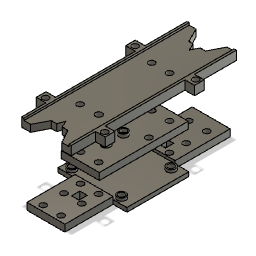
self balancing robot (Autodesk Fusion 360 design; units mm, degrees)
Autodesk Fusion 360 part; units mm, degrees
sketch "Sketch1" plane through (0, 0, 0) normal (0, 1, 0) x (1, 0, 0)
  circle A0 centre (-15, 25) radius 2.25
  circle A1 centre (-2, 25) radius 2.25
  circle A2 centre (-15, 40) radius 2.25
  circle A3 centre (-2, 40) radius 2.25
  line L0 (-11.7906, 20.4996) -> (-6.4075, 20.4996)
  line L1 (-6.4075, 20.4996) -> (-6.4075, 14.4996)
  line L2 (-6.4075, 14.4996) -> (-11.7906, 14.4996)
  line L3 (-11.7906, 14.4996) -> (-11.7906, 20.4996)
  circle A4 centre (-15, 12.9146) radius 2.25
  circle A5 centre (-2, 12.9014) radius 2.25
  circle A6 centre (7.0301, 5.1014) radius 2.25
  circle A7 centre (-28.9699, 5) radius 2.25
  circle A8 centre (-28.9697, -31) radius 2.25
  circle A9 centre (7.0301, -30.8986) radius 2.25
  circle A10 centre (-1.841, -50.8854) radius 2.25
  circle A11 centre (-14.841, -50.8854) radius 2.25
  line L4 (-10.4335, -49.7263) -> (-10.4335, -43.7263)
  circle A12 centre (-14.841, -38.8) radius 2.25
  circle A13 centre (-14.841, -65.8854) radius 2.25
  circle A14 centre (-1.841, -65.8854) radius 2.25
  circle A15 centre (-1.841, -38.6986) radius 2.25
  line L5 (-5.0503, -43.7263) -> (-5.0503, -49.7263)
  line L6 (-10.4335, -43.7263) -> (-5.0503, -43.7263)
  line L7 (-5.0503, -49.7263) -> (-10.4335, -49.7263)
  line L8 (-35, 50) -> (15, 50)
  line L9 (15, 50) -> (15, -70)
  line L10 (15, -70) -> (-35, -70)
  line L11 (-35, -70) -> (-35, 50)
  line L12 (5, 50) -> (5, 10)
  line L13 (5, 10) -> (15, 10)
  line L14 (-22.5777, 50) -> (-22.5777, 10)
  line L15 (-22.5777, 10) -> (-35, 10)
  line L16 (-22.5777, -70) -> (-22.5777, -35)
  line L17 (-22.5777, -35) -> (-35, -35)
  line L18 (5, -70) -> (5, -35)
  line L19 (5, -35) -> (15, -35)
  dimension "d1" = 4.5
  dimension "d2" = 4.5
  dimension "d3" = 4.5
  dimension "d4" = 4.5
  dimension "d5" = 15
  dimension "d6" = 13
  dimension "d7" = 13
  dimension "d9" = 6
  dimension "d10" = 4.5
  dimension "d11" = 4.5
  dimension "d15" = 4.5
  dimension "d16" = 4.5
  dimension "d17" = 4.5
  dimension "d18" = 4.5
  dimension "d19" = 36
  dimension "d20" = 36
  dimension "d21" = 36
  dimension "d22" = 36
  dimension "d23" = 4.5
  dimension "d24" = 4.5
  dimension "d25" = 4.5
  dimension "d26" = 4.5
  dimension "d27" = 15
  dimension "d28" = 13
  dimension "d29" = 13
  dimension "d30" = 6
  dimension "d31" = 4.5
  dimension "d32" = 4.5
  dimension "d33" = 7.8
  dimension "d34" = 7.8
  dimension "d35" = 13
  dimension "d36" = 13
  dimension "d37" = 12.0986
  dimension "d38" = 12.0854
  dimension "d39" = 7.9146
  dimension "d40" = 7.8
  dimension "d41" = 50
  dimension "d42" = 120
  dimension "d43" = 51.7146
  dimension "d44" = 51.6
  constraint horizontal L0
  constraint vertical L1
  constraint horizontal L2
  constraint vertical L3
  constraint horizontal L8
  constraint vertical L9
  constraint horizontal L10
  constraint vertical L11
  constraint coincident L8 L12.start
  constraint perpendicular L8 L12
  constraint coincident L9 L13.end
  constraint perpendicular L9 L13
  constraint coincident L8 L14.start
  constraint perpendicular L8 L14
  constraint coincident L11 L15.end
  constraint perpendicular L11 L15
  constraint coincident L10 L16.start
  constraint perpendicular L10 L16
  constraint coincident L11 L17.end
  constraint perpendicular L11 L17
  constraint perpendicular L13 L18
  constraint coincident L9 L19.end
  constraint perpendicular L9 L19
  measures "d1" diameter of A0
  measures "d2" diameter of A1
  measures "d3" diameter of A2
  measures "d4" diameter of A3
  measures "d5" distance of A0.centre A2.centre
  measures "d6" distance of A2.centre A3.centre
  measures "d7" distance of A0.centre A1.centre
  measures "d9" distance of L0.start L2.end
  measures "d10" diameter of A4
  measures "d11" diameter of A5
  measures "d15" diameter of A6
  measures "d16" diameter of A7
  measures "d17" diameter of A8
  measures "d18" diameter of A9
  measures "d19" horizontal distance of A6.centre A7.centre
  measures "d20" vertical distance of A7.centre A8.centre
  measures "d21" distance of A6.centre A9.centre
  measures "d22" distance of A8.centre A9.centre
  measures "d23" diameter of A10
  measures "d24" diameter of A11
  measures "d25" diameter of A14
  measures "d26" diameter of A13
  measures "d27" distance of A14.centre A10.centre
  measures "d28" distance of A14.centre A13.centre
  measures "d29" distance of A11.centre A10.centre
  measures "d30" distance of L5.end L5.start
  measures "d31" diameter of A15
  measures "d32" diameter of A12
  measures "d33" vertical distance of A5.centre A6.centre
  measures "d34" vertical distance of A9.centre A15.centre
  measures "d35" horizontal distance of A4.centre A5.centre
  measures "d36" horizontal distance of A15.centre A12.centre
  measures "d37" distance of A1.centre A5.centre
  measures "d38" distance of A12.centre A11.centre
  measures "d39" vertical distance of A4.centre A7.centre
  measures "d40" vertical distance of A8.centre A12.centre
  measures "d41" distance of L8.start L8.end
  measures "d42" distance of L8.start L10.end
  measures "d43" vertical distance of A4.centre A12.centre
  measures "d44" vertical distance of A5.centre A15.centre
extrude "Extrude1" add sketch "Sketch1" along normal blind 5 contours L8 L9 L10 L11 L12 L13 L14 L15 L16 L17 L18 L19 makes body 1
sketch "Sketch2" plane through (0, 5, 0) normal (0, 1, 0) x (-1, 0, 0)
  circle A0 centre (14.841, 65.8854) radius 2.25
  circle A1 centre (1.841, 38.6986) radius 2.25
  circle A2 centre (1.841, 65.8854) radius 2.25
  circle A3 centre (14.841, 38.8) radius 2.25
  line L0 (5.0503, 43.7263) -> (5.0503, 49.7263)
  line L1 (5.0503, 49.7263) -> (10.4335, 49.7263)
  line L2 (10.4335, 49.7263) -> (10.4335, 43.7263)
  line L3 (10.4335, 43.7263) -> (5.0503, 43.7263)
  circle A4 centre (-7.0301, -5.1014) radius 2.25
  circle A5 centre (28.9699, -5) radius 2.25
  circle A6 centre (28.9697, 31) radius 2.25
  circle A7 centre (-7.0301, 30.8986) radius 2.25
  circle A8 centre (1.841, 50.8854) radius 2.25
  circle A9 centre (14.841, 50.8854) radius 2.25
  circle A10 centre (2, -12.9014) radius 2.25
  circle A11 centre (15, -12.9146) radius 2.25
  circle A12 centre (2, -40) radius 2.25
  line L4 (6.4075, -14.4996) -> (11.7906, -14.4996)
  line L5 (11.7906, -14.4996) -> (11.7906, -20.4996)
  line L6 (11.7906, -20.4996) -> (6.4075, -20.4996)
  line L7 (6.4075, -20.4996) -> (6.4075, -14.4996)
  circle A13 centre (15, -40) radius 2.25
  circle A14 centre (2, -25) radius 2.25
  circle A15 centre (15, -25) radius 2.25
  line L8 (-5, 70) -> (-5, 35)
  line L9 (-5, 35) -> (-15, 35)
  line L10 (-15, 35) -> (-15, -10)
  line L11 (-15, -10) -> (-5, -10)
  line L12 (-5, -10) -> (-5, -50)
  line L13 (-5, -50) -> (22.5777, -50)
  line L14 (22.5777, -50) -> (22.5777, -10)
  line L15 (22.5777, -10) -> (35, -10)
  line L16 (35, -10) -> (35, 35)
  line L17 (35, 35) -> (22.5777, 35)
  line L18 (22.5777, 35) -> (22.5777, 70)
  line L19 (22.5777, 70) -> (-5, 70)
  line L20 (35, -10) -> (-15, -10)
  line L21 (-15, -10) -> (-15, 35)
  line L22 (-15, 35) -> (35, 35)
  line L23 (35, 35) -> (35, -10)
  circle A16 centre (28.9699, -5) radius 2.8072
  circle A17 centre (-7.0301, -5.1014) radius 3.2495
  circle A18 centre (-7.0301, 30.8986) radius 3.07
  circle A19 centre (28.9697, 31) radius 3.1528
  constraint horizontal L20
  constraint vertical L21
  constraint horizontal L22
  constraint vertical L23
  constraint coincident L9.end L10.start
  constraint coincident L15.end L16.start
  constraint concentric A5 A16
  constraint concentric A4 A17
  constraint concentric A7 A18
  constraint concentric A6 A19
extrude "Extrude2" cut sketch "Sketch2" against normal blind 2 contours L9 L10 L11 L15 L16 L17 L20 L21 L22 L23 bodies 1
sketch "Sketch3" plane through (0, 0, 0) normal (0, 0, 1) x (1, 0, 0)
sketch "Sketch4" plane through (0, 0, 0) normal (0, 1, 0) x (1, 0, 0)
  circle A0 centre (-15, 13) radius 2.25
  circle A1 centre (-2, 13) radius 2.25
  circle A2 centre (-14.819, -38.8151) radius 2.25
  circle A3 centre (-1.741, -38.7383) radius 2.25
  line L0 (-22.7552, 19.5423) -> (5, 19.5423)
  line L1 (5, 19.5423) -> (5, -45)
  line L2 (5, -45) -> (-22.7552, -45)
  line L3 (-22.7552, -45) -> (-22.7552, 19.5423)
  dimension "d49" = 4.5
  dimension "d50" = 4.5
  dimension "d51" = 4.5
  dimension "d52" = 4.5
  constraint horizontal L0
  constraint vertical L1
  constraint horizontal L2
  constraint vertical L3
  measures "d49" diameter of A0
  measures "d50" diameter of A1
  measures "d51" diameter of A2
  measures "d52" diameter of A3
extrude "Extrude3" add sketch "Sketch4" along normal blind 5 separate body makes body 2
move_body "Move1" bodies 2 to x (1, 0, 0) y (0, 1, 0) z (0, 0, 1) at (0, 20, 0)
sketch "Sketch5" plane through (0, 25, 0) normal (0, 1, 0) x (-1, 0, 0)
  circle A0 centre (14.819, 38.8151) radius 2.25
  circle A1 centre (1.741, 38.7383) radius 2.25
  circle A2 centre (2, -13) radius 2.25
  circle A3 centre (15, -13) radius 2.25
  line L0 (22.7552, 45) -> (-5, 45)
  line L1 (-5, 45) -> (-5, -19.5423)
  line L2 (-5, -19.5423) -> (22.7552, -19.5423)
  line L3 (22.7552, -19.5423) -> (22.7552, 45)
  circle A4 centre (10, 25) radius 2.25
  circle A5 centre (10, 12.5) radius 2.25
  circle A6 centre (10, 12.5) radius 3
  circle A7 centre (10, 25) radius 3
  circle A8 centre (-1, 5) radius 2.25
  dimension "d55" = 4.5
  dimension "d56" = 4.5
  dimension "d57" = 12.5
  dimension "d58" = 6
  dimension "d59" = 6
  dimension "d60" = 4.5
  constraint concentric A5 A6
  constraint concentric A4 A7
  measures "d55" diameter of A4
  measures "d56" diameter of A5
  measures "d57" distance of A4.centre A5.centre
  measures "d58" diameter of A6
  measures "d59" diameter of A7
  measures "d60" diameter of A8
extrude "Extrude4" add sketch "Sketch5" along normal blind 2.5 contours A6 | A7 bodies 2
extrude "Extrude5" cut sketch "Sketch5" against normal blind 5 contours A8 bodies 2
extrude "Extrude6" add sketch "Sketch5" against normal blind 5 contours A8 bodies 2
extrude "Extrude7" cut sketch "Sketch5" against normal blind 7 contours A8 bodies 2
sketch "Sketch6" plane through (0, 0, 0) normal (0, 1, 0) x (1, 0, 0)
  line L0 (-26.7355, 50.3207) -> (9.2645, 50.3207)
  line L1 (9.2645, 50.3207) -> (9.2645, -69.6793)
  line L2 (9.2645, -69.6793) -> (-26.7355, -69.6793)
  line L3 (-26.7355, -69.6793) -> (-26.7355, 50.3207)
  circle A0 centre (-14.9855, 13.0272) radius 2.25
  circle A1 centre (-2.0435, 13.0272) radius 2.25
  circle A2 centre (-15, -39) radius 2.25
  circle A3 centre (-1.6771, -38.6684) radius 2.4279
  line L4 (9.2645, 19.8475) -> (16.2645, 19.8475)
  line L5 (16.2645, 19.8475) -> (16.2645, 12.8475)
  line L6 (16.2645, 12.8475) -> (9.2645, 12.8475)
  line L7 (9.2645, 12.8475) -> (9.2645, 19.8475)
  line L8 (9.2645, -45.0475) -> (16.2645, -45.0475)
  line L9 (16.2645, -45.0475) -> (16.2645, -52.0475)
  line L10 (16.2645, -52.0475) -> (9.2645, -52.0475)
  line L11 (9.2645, -52.0475) -> (9.2645, -45.0475)
  line L12 (-26.7355, 19.8475) -> (-33.7355, 19.8475)
  line L13 (-33.7355, 19.8475) -> (-33.7355, 12.8475)
  line L14 (-33.7355, 12.8475) -> (-26.7355, 12.8475)
  line L15 (-26.7355, 12.8475) -> (-26.7355, 19.8475)
  line L16 (-26.7355, -45.0475) -> (-33.7355, -45.0475)
  line L17 (-33.7355, -45.0475) -> (-33.7355, -52.0475)
  line L18 (-33.7355, -52.0475) -> (-26.7355, -52.0475)
  line L19 (-26.7355, -52.0475) -> (-26.7355, -45.0475)
  circle A4 centre (-30, 16) radius 2.25
  circle A5 centre (13, 17) radius 2.25
  circle A6 centre (13, -49) radius 2.25
  circle A7 centre (-30, -49) radius 2.25
  line L20 (-20.1067, 50.3207) -> (-15, 40)
  line L21 (-15, 40) -> (-11.9429, 40)
  line L22 (-11.9429, 40) -> (-9.3767, 34.8138)
  line L23 (-9.3767, 34.8138) -> (-6.6947, 40)
  line L24 (-6.6947, 40) -> (-2.9044, 40)
  line L25 (-2.9044, 40) -> (2.4328, 50.3207)
  line L26 (-20.284, -69.6793) -> (-15.1632, -59.7773)
  line L27 (-15.1632, -59.7773) -> (-15.2822, -59.7773)
  line L28 (-9.3767, 34.8138) -> (-9.3767, -54.8804) construction
  line L29 (2.4328, 50.3207) -> (2.4328, -69.6793) construction
  line L30 (-2.9044, 40) -> (-2.9044, -60) construction
  line L31 (-15, 40) -> (-15.2227, -59.7773) construction
  line L32 (-15.2822, -59.7773) -> (-11.2248, -59.7773)
  line L33 (-11.2248, -59.7773) -> (-9.3767, -54.8804)
  line L34 (-9.3767, -54.8804) -> (-7.1721, -59.7773)
  line L35 (-7.1721, -59.7773) -> (-2.9044, -60)
  line L36 (-2.9044, -60) -> (2.4328, -69.6793)
  dimension "d69" = 36
  dimension "d70" = 120
  dimension "d71" = 4.5
  dimension "d72" = 4.5
  dimension "d73" = 4.5
  dimension "d74" = 7
  dimension "d75" = 7
  dimension "d76" = 7
  dimension "d77" = 7
  dimension "d78" = 7
  dimension "d79" = 7
  dimension "d80" = 7
  dimension "d81" = 7
  dimension "d82" = 4.5
  dimension "d83" = 4.5
  dimension "d84" = 4.5
  dimension "d85" = 4.5
  constraint horizontal L0
  constraint vertical L1
  constraint horizontal L2
  constraint vertical L3
  constraint horizontal L4
  constraint vertical L5
  constraint horizontal L6
  constraint vertical L7
  constraint coincident L1 L4.start
  constraint horizontal L8
  constraint vertical L9
  constraint horizontal L10
  constraint vertical L11
  constraint coincident L1 L8.start
  constraint horizontal L12
  constraint vertical L13
  constraint horizontal L14
  constraint vertical L15
  constraint coincident L3 L12.start
  constraint horizontal L16
  constraint vertical L17
  constraint horizontal L18
  constraint vertical L19
  constraint coincident L3 L16.start
  constraint coincident L0 L20.start
  constraint parallel L0 L21
  constraint parallel L20 L22
  constraint parallel L21 L24
  constraint coincident L0 L25.end
  constraint parallel L23 L25
  constraint coincident L2 L26.start
  constraint parallel L25 L26
  constraint parallel L2 L27
  constraint vertical L28
  constraint coincident L2 L29.end
  constraint perpendicular L2 L29
  constraint perpendicular L24 L30
  constraint midpoint L27 L31.end
  measures "d69" distance of L0.start L0.end
  measures "d70" distance of L0.start L2.end
  measures "d71" diameter of A0
  measures "d72" diameter of A1
  measures "d73" diameter of A2
  measures "d74" distance of L4.start L4.end
  measures "d75" distance of L4.start L6.end
  measures "d76" distance of L8.start L8.end
  measures "d77" distance of L8.start L10.end
  measures "d78" distance of L12.start L12.end
  measures "d79" distance of L12.start L14.end
  measures "d80" distance of L16.start L16.end
  measures "d81" distance of L16.start L18.end
  measures "d82" diameter of A4
  measures "d83" diameter of A5
  measures "d84" diameter of A6
  measures "d85" diameter of A7
extrude "Extrude8" add sketch "Sketch6" along normal blind 5 separate body contours L0 L1 L2 L3 L7 L11 L15 L19 L20 L21 L22 L23 L24 L25 L26 L32 L33 L34 L35 L36 | L3 L12 L13 L14 L15 | L3 L16 L17 L18 L19 | L1 L4 L5 L6 L7 | L1 L8 L9 L10 L11 makes body 3
sketch "Sketch7" plane through (0, 5, 0) normal (0, 1, 0) x (-1, 0, 0)
  circle A0 centre (30, 49) radius 2.25
  circle A1 centre (-13, -17) radius 2.25
  circle A2 centre (15, 39) radius 2.25
  circle A3 centre (-13, 49) radius 2.25
  circle A4 centre (1.6771, 38.6684) radius 2.4279
  circle A5 centre (30, -16) radius 2.25
  circle A6 centre (2.0435, -13.0272) radius 2.25
  circle A7 centre (14.9855, -13.0272) radius 2.25
  line L0 (20.284, 69.6793) -> (15.1632, 59.7773)
  line L1 (15.1632, 59.7773) -> (11.2248, 59.7773)
  line L2 (11.2248, 59.7773) -> (9.3767, 54.8804)
  line L3 (9.3767, 54.8804) -> (7.1721, 59.7773)
  line L4 (7.1721, 59.7773) -> (2.9044, 60)
  line L5 (2.9044, 60) -> (-2.4328, 69.6793)
  line L6 (-2.4328, 69.6793) -> (-9.2645, 69.6793)
  line L7 (-9.2645, 69.6793) -> (-9.2645, 52.0475)
  line L8 (-9.2645, 52.0475) -> (-16.2645, 52.0475)
  line L9 (-16.2645, 52.0475) -> (-16.2645, 45.0475)
  line L10 (-16.2645, 45.0475) -> (-9.2645, 45.0475)
  line L11 (-9.2645, 45.0475) -> (-9.2645, -12.8475)
  line L12 (-9.2645, -12.8475) -> (-16.2645, -12.8475)
  line L13 (-16.2645, -12.8475) -> (-16.2645, -19.8475)
  line L14 (-16.2645, -19.8475) -> (-9.2645, -19.8475)
  line L15 (-9.2645, -19.8475) -> (-9.2645, -50.3207)
  line L16 (-9.2645, -50.3207) -> (-2.4328, -50.3207)
  line L17 (-2.4328, -50.3207) -> (2.9044, -40)
  line L18 (2.9044, -40) -> (6.6947, -40)
  line L19 (6.6947, -40) -> (9.3767, -34.8138)
  line L20 (9.3767, -34.8138) -> (11.9429, -40)
  line L21 (11.9429, -40) -> (15, -40)
  line L22 (15, -40) -> (20.1067, -50.3207)
  line L23 (20.1067, -50.3207) -> (26.7355, -50.3207)
  line L24 (26.7355, -50.3207) -> (26.7355, -19.8475)
  line L25 (26.7355, -19.8475) -> (33.7355, -19.8475)
  line L26 (33.7355, -19.8475) -> (33.7355, -12.8475)
  line L27 (33.7355, -12.8475) -> (26.7355, -12.8475)
  line L28 (26.7355, -12.8475) -> (26.7355, 45.0475)
  line L29 (26.7355, 45.0475) -> (33.7355, 45.0475)
  line L30 (33.7355, 45.0475) -> (33.7355, 52.0475)
  line L31 (33.7355, 52.0475) -> (26.7355, 52.0475)
  line L32 (26.7355, 52.0475) -> (26.7355, 69.6793)
  line L33 (26.7355, 69.6793) -> (20.284, 69.6793)
  line L34 (-7.5721, -50.3207) -> (-7.5721, 69.6793)
  line L35 (25.1065, -50.3207) -> (25.1065, 69.6793)
  constraint coincident L16 L34.start
  constraint coincident L6 L34.end
  constraint perpendicular L6 L34
  constraint coincident L23 L35.start
  constraint coincident L33 L35.end
  constraint perpendicular L33 L35
extrude "Extrude9" add sketch "Sketch7" along normal blind 1.5 contours L23 L24 L25 L26 L27 L28 L29 L30 L31 L32 L33 L35 | L6 L7 L8 L9 L10 L11 L12 L13 L14 L15 L16 L34 bodies 3
move_body "Move2" bodies 3 to x (1, 0, 0) y (0, 1, 0) z (0, 0, 1) at (0, 50, 0)
